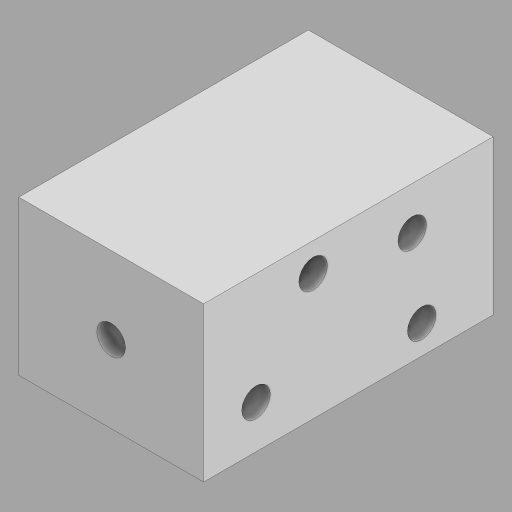
# Autodesk Inventor part: Solinoyd_telo
Saved by Autodesk Inventor 2024.2 (Build 282272000, 272)
## iProperties
Created: 2023-12-22
Part Number: Solinoyd_telo
Material: Типовые
Document SubType Name: Modeling
Designer: Fedor Orlov
Density: 1 g/cm^3
Appearance: По умолчанию
Author: Fedor Orlov
Autodesk Inventor part; units mm, degrees
ref_plane "YZ Plane" through (0, 0, 0) normal (1, 0, 0) x (0, 1, 0)
ref_plane "XZ Plane" through (0, 0, 0) normal (0, 1, 0) x (-1, 0, 0)
ref_plane "XY Plane" through (0, 0, 0) normal (0, 0, 1) x (1, 0, 0)
sketch "Эскиз1" plane through (0, 0, 0) normal (0, 1, 0) x (-1, 0, 0)
  line L0 (-9.7, -15.2) -> (9.7, -15.2)
  line L1 (9.7, -15.2) -> (9.7, 15.2)
  line L2 (9.7, 15.2) -> (-9.7, 15.2)
  line L3 (-9.7, 15.2) -> (-9.7, -15.2)
  line L4 (-9.7, -15.2) -> (9.7, 15.2) construction
  line L5 (9.7, -15.2) -> (-9.7, 15.2) construction
  point P0 (0, 0)
  dimension "d0" = 30.4
  dimension "d1" = 19.4
  constraints: 12 end point, 2 midpoint, 2 parallel, 1 horizontal, 1 perpendicular
  measures "d0" distance of L0.end L1.end
  measures "d1" distance of L1.end L2.end
extrude "Выдавливание1" add sketch "Эскиз1" along normal blind 16.2
sketch "Эскиз2" plane through (9.7, 0, -15.2) normal (0, 0, -1) x (-1, 0, 0)
  line L0 (19.4, 16.2) -> (0, 16.2) projected
  line L1 (19.4, 0) -> (19.4, 16.2) projected
  line L2 (0, 16.2) -> (19.4, 0) construction
  line L3 (19.4, 0) -> (0, 0) projected
  line L4 (19.4, 16.2) -> (0, 0) construction
  circle A0 centre (9.7, 8.1) radius 1.5
  point P0 (9.7, 0)
  dimension "d4" = 3
  constraints: 4 end point, 1 centre point, 1 midpoint
  measures "d4" diameter of A0
extrude "Выдавливание2" cut sketch "Эскиз2" against normal through all
sketch "Эскиз3" plane through (9.7, 0, 15.2) normal (1, 0, 0) x (0, 0, -1)
  circle A0 centre (21.9, 11.7) radius 1.5
  line L0 (0, 16.2) -> (30.4, 16.2) projected
  line L1 (30.4, 0) -> (30.4, 16.2) projected
  circle A1 centre (5.5, 4.5) radius 1.5
  circle A2 centre (22.9, 3) radius 1.5
  circle A3 centre (11.5, 13.2) radius 1.5
  line L2 (0, 0) -> (30.4, 0) projected
  line L3 (0, 0) -> (0, 16.2) projected
  point P0 (15.2, 0)
  dimension "d7" = 3
  dimension "d8" = 4.5
  dimension "d9" = 8.5
  dimension "d10" = 3
  dimension "d11" = 3
  dimension "d12" = 3
  dimension "d13" = 4.5
  dimension "d14" = 3
  dimension "d15" = 3
  dimension "d16" = 7.5
  dimension "d17" = 5.5
  dimension "d18" = 11.5
  constraints: 4 centre point
  measures "d7" diameter of A0
  measures "d8" distance from line of L0 A0.centre
  measures "d9" distance from line of L1 A0.centre
  measures "d10" diameter of A1
  measures "d11" diameter of A2
  measures "d12" diameter of A3
  measures "d13" distance from line of L2 A1.centre
  measures "d14" distance from line of L2 A2.centre
  measures "d15" distance from line of L0 A3.centre
  measures "d16" distance from line of L1 A2.centre
  measures "d17" distance from line of L3 A1.centre
  measures "d18" distance from line of L3 A3.centre
extrude "Выдавливание3" cut sketch "Эскиз3" against normal blind 3.5 contours A0 | A1 | A2 | A3
sketch "Эскиз4" plane through (9.7, 0, -15.2) normal (0, 0, -1) x (-1, 0, 0)
  line L0 (16.2554, 14.2612) -> (16.2554, 1.9388) construction
  line L1 (16.2554, 1.9388) -> (12.5446, 1.9388) construction
  line L2 (12.5446, 1.9388) -> (12.5446, 14.2612) construction
  line L3 (12.5446, 14.2612) -> (16.2554, 14.2612) construction
  line L4 (16.2554, 1.9388) -> (12.5446, 14.2612) construction
  line L5 (16.2554, 14.2612) -> (12.5446, 1.9388) construction
  circle A0 centre (9.7, 8.1) radius 1.5 projected
  line L6 (0, 0) -> (0, 16.2) projected
  line L7 (0, 8.1) -> (19.4, 8.1) construction
  line L8 (19.4, 0) -> (19.4, 16.2) projected
  line L9 (13.2074, 11.7393) -> (13.2074, 12.1444)
  line L10 (13.2074, 12.1444) -> (15.8947, 12.1444)
  line L11 (15.8947, 12.1444) -> (15.8947, 13.5473)
  line L12 (15.8947, 13.5473) -> (13.2074, 13.5473)
  line L13 (13.2074, 13.5473) -> (13.2074, 13.9524)
  line L14 (13.2074, 13.9524) -> (16.2554, 13.9524)
  line L15 (16.2554, 13.9524) -> (16.2554, 11.7393)
  line L16 (16.2554, 11.7393) -> (13.2074, 11.7393)
  spline S0 degree 2 poles (13.1555, 10.1585) (13.1555, 10.7068) (13.7705, 11.3095) (14.3386, 11.3095) knots 0 0 0 1 2 2 2
  spline S1 degree 2 poles (14.3386, 11.3095) (14.8969, 11.3095) (15.5588, 10.7241) (15.5588, 10.2523) knots 0 0 0 1 2 2 2
  spline S2 degree 2 poles (15.5588, 10.2523) (15.5588, 10.0399) (15.4353, 9.7114) (15.3044, 9.5904) knots 0 0 0 1 2 2 2
  spline S3 degree 2 poles (15.3044, 9.5904) (15.1735, 9.4669) (14.7956, 9.336) (14.5214, 9.336) knots 0 0 0 1 2 2 2
  line L17 (14.5214, 9.336) -> (14.3115, 9.336)
  line L18 (14.3115, 9.336) -> (14.3115, 10.9193)
  spline S4 degree 2 poles (14.3115, 10.9193) (13.9138, 10.9193) (13.4914, 10.5191) (13.4914, 10.1634) knots 0 0 0 1 2 2 2
  spline S5 degree 2 poles (13.4914, 10.1634) (13.4914, 10.0375) (13.5482, 9.7929) (13.5927, 9.6941) knots 0 0 0 1 2 2 2
  spline S6 degree 2 poles (13.5927, 9.6941) (13.6421, 9.5904) (13.7285, 9.4471) (13.7681, 9.4002) knots 0 0 0 1 2 2 2
  line L19 (13.7681, 9.4002) -> (13.7681, 9.378)
  line L20 (13.7681, 9.378) -> (13.3482, 9.378)
  spline S7 degree 2 poles (13.3482, 9.378) (13.321, 9.4447) (13.2419, 9.6472) (13.2197, 9.7262) knots 0 0 0 1 2 2 2
  spline S8 degree 2 poles (13.2197, 9.7262) (13.1876, 9.8374) (13.1555, 10.0202) (13.1555, 10.1585) knots 0 0 0 1 2 2 2
  spline S9 degree 2 poles (14.6054, 9.7114) (14.761, 9.7164) (14.9882, 9.7806) (15.0648, 9.8423) knots 0 0 0 1 2 2 2
  spline S10 degree 2 poles (15.0648, 9.8423) (15.1513, 9.909) (15.2427, 10.119) (15.2427, 10.2746) knots 0 0 0 1 2 2 2
  spline S11 degree 2 poles (15.2427, 10.2746) (15.2427, 10.4277) (15.1513, 10.6426) (15.0623, 10.7315) knots 0 0 0 1 2 2 2
  spline S12 degree 2 poles (15.0623, 10.7315) (14.971, 10.818) (14.7511, 10.9069) (14.6054, 10.9193) knots 0 0 0 1 2 2 2
  line L21 (14.6054, 10.9193) -> (14.6054, 9.7114)
  line L22 (13.2074, 7.1426) -> (13.2074, 7.5279)
  line L23 (13.2074, 7.5279) -> (15.1636, 7.5279)
  line L24 (15.1636, 7.5279) -> (15.1636, 8.5604)
  line L25 (15.1636, 8.5604) -> (13.2074, 8.5604)
  line L26 (13.2074, 8.5604) -> (13.2074, 8.9457)
  line L27 (13.2074, 8.9457) -> (15.4946, 8.9457)
  line L28 (15.4946, 8.9457) -> (15.4946, 7.1426)
  line L29 (15.4946, 7.1426) -> (13.2074, 7.1426)
  spline S13 degree 2 poles (13.1555, 5.5914) (13.1555, 6.1398) (13.7705, 6.7425) (14.3386, 6.7425) knots 0 0 0 1 2 2 2
  spline S14 degree 2 poles (14.3386, 6.7425) (14.8969, 6.7425) (15.5588, 6.1571) (15.5588, 5.6853) knots 0 0 0 1 2 2 2
  spline S15 degree 2 poles (15.5588, 5.6853) (15.5588, 5.4729) (15.4353, 5.1444) (15.3044, 5.0233) knots 0 0 0 1 2 2 2
  spline S16 degree 2 poles (15.3044, 5.0233) (15.1735, 4.8998) (14.7956, 4.7689) (14.5214, 4.7689) knots 0 0 0 1 2 2 2
  line L30 (14.5214, 4.7689) -> (14.3115, 4.7689)
  line L31 (14.3115, 4.7689) -> (14.3115, 6.3522)
  spline S17 degree 2 poles (14.3115, 6.3522) (13.9138, 6.3522) (13.4914, 5.952) (13.4914, 5.5964) knots 0 0 0 1 2 2 2
  spline S18 degree 2 poles (13.4914, 5.5964) (13.4914, 5.4704) (13.5482, 5.2259) (13.5927, 5.1271) knots 0 0 0 1 2 2 2
  spline S19 degree 2 poles (13.5927, 5.1271) (13.6421, 5.0233) (13.7285, 4.8801) (13.7681, 4.8331) knots 0 0 0 1 2 2 2
  line L32 (13.7681, 4.8331) -> (13.7681, 4.8109)
  line L33 (13.7681, 4.8109) -> (13.3482, 4.8109)
  spline S20 degree 2 poles (13.3482, 4.8109) (13.321, 4.8776) (13.2419, 5.0801) (13.2197, 5.1592) knots 0 0 0 1 2 2 2
  spline S21 degree 2 poles (13.2197, 5.1592) (13.1876, 5.2703) (13.1555, 5.4531) (13.1555, 5.5914) knots 0 0 0 1 2 2 2
  spline S22 degree 2 poles (14.6054, 5.1444) (14.761, 5.1493) (14.9882, 5.2135) (15.0648, 5.2753) knots 0 0 0 1 2 2 2
  spline S23 degree 2 poles (15.0648, 5.2753) (15.1513, 5.342) (15.2427, 5.5519) (15.2427, 5.7075) knots 0 0 0 1 2 2 2
  spline S24 degree 2 poles (15.2427, 5.7075) (15.2427, 5.8607) (15.1513, 6.0755) (15.0623, 6.1645) knots 0 0 0 1 2 2 2
  spline S25 degree 2 poles (15.0623, 6.1645) (14.971, 6.2509) (14.7511, 6.3398) (14.6054, 6.3522) knots 0 0 0 1 2 2 2
  line L34 (14.6054, 6.3522) -> (14.6054, 5.1444)
  line L35 (12.659, 2.4199) -> (12.659, 2.7781)
  line L36 (12.659, 2.7781) -> (13.2123, 2.7781)
  line L37 (13.2123, 2.7781) -> (13.2123, 4.2823)
  line L38 (13.2123, 4.2823) -> (12.659, 4.2823)
  line L39 (12.659, 4.2823) -> (12.659, 4.6405)
  line L40 (12.659, 4.6405) -> (13.5359, 4.6405)
  line L41 (13.5359, 4.6405) -> (13.5359, 4.4898)
  spline S26 degree 2 poles (13.5359, 4.4898) (13.8545, 4.2947) (14.8845, 4.0477) (15.4946, 4.0477) knots 0 0 0 1 2 2 2
  line L42 (15.4946, 4.0477) -> (15.4946, 2.6472)
  line L43 (15.4946, 2.6472) -> (13.5359, 2.6472)
  line L44 (13.5359, 2.6472) -> (13.5359, 2.4199)
  line L45 (13.5359, 2.4199) -> (12.659, 2.4199)
  line L46 (13.5359, 3.0325) -> (15.171, 3.0325)
  line L47 (15.171, 3.0325) -> (15.171, 3.6846)
  spline S27 degree 2 poles (15.171, 3.6846) (14.6597, 3.7117) (13.815, 3.939) (13.5359, 4.1119) knots 0 0 0 1 2 2 2
  line L48 (13.5359, 4.1119) -> (13.5359, 3.0325)
  point P0 (9.7, 0)
  point P1 (14.4, 8.1)
  point P2 (14.4, 8.1)
  dimension "d21" = 5
  constraints: 6 end point, 4 midpoint, 1 point on line, 2 other
  measures "d21" distance from line of L8 point (14.4, 8.1)
extrude "Выдавливание4" cut sketch "Эскиз4" against normal blind 0.2 contours L9 L10 L11 L12 L13 L14 L15 L16 | S0 S1 S2 S3 L17 L18 S4 S5 S6 L19 L20 S7 S8 | L22 L23 L24 L25 L26 L27 L28 L29 | S13 S14 S15 S16 L30 L31 S17 S18 S19 L32 L33 S20 S21 | L35 L36 L37 L38 L39 L40 L41 S26 L42 L43 L44 L45
sketch "Эскиз5" plane through (-9.7, 0, -15.2) normal (-1, 0, 0) x (0, 0, 1)
  line L0 (9.6722, 9.7186) -> (20.6663, 9.7186) construction
  line L1 (20.6663, 9.7186) -> (20.6663, 6.5249) construction
  line L2 (20.6663, 6.5249) -> (9.6722, 6.5249) construction
  line L3 (9.6722, 6.5249) -> (9.6722, 9.7186) construction
  line L4 (20.6663, 9.7186) -> (9.6722, 6.5249) construction
  line L5 (20.6663, 6.5249) -> (9.6722, 9.7186) construction
  line L6 (30.4, 0) -> (30.4, 16.2) projected
  line L7 (0, 0) -> (0, 16.2) projected
  line L8 (30.4, 16.2) -> (0, 0) construction
  line L9 (0, 16.2) -> (30.4, 16.2) projected
  line L10 (0, 0) -> (30.4, 0) projected
  line L11 (0, 16.2) -> (30.4, 0) construction
  spline S0 degree 2 poles (11.7446, 8.0587) (11.7446, 7.8933) (11.6186, 7.6364) (11.5075, 7.5524) knots 0 0 0 1 2 2 2
  spline S1 degree 2 poles (11.5075, 7.5524) (11.3691, 7.4437) (11.0629, 7.3671) (10.8504, 7.3671) knots 0 0 0 1 2 2 2
  line L12 (10.8504, 7.3671) -> (9.9513, 7.3671)
  line L13 (9.9513, 7.3671) -> (9.9513, 9.6544)
  line L14 (9.9513, 9.6544) -> (10.7912, 9.6544)
  spline S2 degree 2 poles (10.7912, 9.6544) (11.0431, 9.6544) (11.2753, 9.6247) (11.3914, 9.5605) knots 0 0 0 1 2 2 2
  spline S3 degree 2 poles (11.3914, 9.5605) (11.5124, 9.4938) (11.626, 9.2765) (11.626, 9.1283) knots 0 0 0 1 2 2 2
  spline S4 degree 2 poles (11.626, 9.1283) (11.626, 8.9652) (11.4457, 8.7034) (11.2975, 8.6318) knots 0 0 0 1 2 2 2
  line L15 (11.2975, 8.6318) -> (11.3074, 8.6194)
  spline S5 degree 2 poles (11.3074, 8.6194) (11.4926, 8.57) (11.7446, 8.2835) (11.7446, 8.0587) knots 0 0 0 1 2 2 2
  spline S6 degree 2 poles (11.3469, 8.0563) (11.3469, 8.1748) (11.2802, 8.3156) (11.1641, 8.37) knots 0 0 0 1 2 2 2
  spline S7 degree 2 poles (11.1641, 8.37) (11.0925, 8.4045) (10.9295, 8.4218) (10.7837, 8.4218) knots 0 0 0 1 2 2 2
  line L16 (10.7837, 8.4218) -> (10.3317, 8.4218)
  line L17 (10.3317, 8.4218) -> (10.3317, 7.6734)
  line L18 (10.3317, 7.6734) -> (10.6652, 7.6734)
  spline S8 degree 2 poles (10.6652, 7.6734) (10.8727, 7.6734) (11.1024, 7.7055) (11.1839, 7.7549) knots 0 0 0 1 2 2 2
  spline S9 degree 2 poles (11.1839, 7.7549) (11.2703, 7.8093) (11.3469, 7.9476) (11.3469, 8.0563) knots 0 0 0 1 2 2 2
  spline S10 degree 2 poles (11.2283, 9.069) (11.2283, 9.148) (11.1765, 9.2616) (11.1147, 9.2938) knots 0 0 0 1 2 2 2
  spline S11 degree 2 poles (11.1147, 9.2938) (11.0406, 9.3333) (10.8578, 9.3481) (10.6973, 9.3481) knots 0 0 0 1 2 2 2
  line L19 (10.6973, 9.3481) -> (10.3317, 9.3481)
  line L20 (10.3317, 9.3481) -> (10.3317, 8.7207)
  line L21 (10.3317, 8.7207) -> (10.7739, 8.7207)
  spline S12 degree 2 poles (10.7739, 8.7207) (10.9147, 8.7207) (11.0332, 8.7479) (11.1048, 8.7899) knots 0 0 0 1 2 2 2
  spline S13 degree 2 poles (11.1048, 8.7899) (11.1715, 8.8319) (11.2283, 8.9702) (11.2283, 9.069) knots 0 0 0 1 2 2 2
  spline S14 degree 2 poles (13.9429, 8.0587) (13.9429, 7.8933) (13.8169, 7.6364) (13.7058, 7.5524) knots 0 0 0 1 2 2 2
  spline S15 degree 2 poles (13.7058, 7.5524) (13.5675, 7.4437) (13.2612, 7.3671) (13.0488, 7.3671) knots 0 0 0 1 2 2 2
  line L22 (13.0488, 7.3671) -> (12.1497, 7.3671)
  line L23 (12.1497, 7.3671) -> (12.1497, 9.6544)
  line L24 (12.1497, 9.6544) -> (12.9895, 9.6544)
  spline S16 degree 2 poles (12.9895, 9.6544) (13.2414, 9.6544) (13.4736, 9.6247) (13.5897, 9.5605) knots 0 0 0 1 2 2 2
  spline S17 degree 2 poles (13.5897, 9.5605) (13.7107, 9.4938) (13.8243, 9.2765) (13.8243, 9.1283) knots 0 0 0 1 2 2 2
  spline S18 degree 2 poles (13.8243, 9.1283) (13.8243, 8.9652) (13.644, 8.7034) (13.4958, 8.6318) knots 0 0 0 1 2 2 2
  line L25 (13.4958, 8.6318) -> (13.5057, 8.6194)
  spline S19 degree 2 poles (13.5057, 8.6194) (13.691, 8.57) (13.9429, 8.2835) (13.9429, 8.0587) knots 0 0 0 1 2 2 2
  spline S20 degree 2 poles (13.5452, 8.0563) (13.5452, 8.1748) (13.4785, 8.3156) (13.3624, 8.37) knots 0 0 0 1 2 2 2
  spline S21 degree 2 poles (13.3624, 8.37) (13.2908, 8.4045) (13.1278, 8.4218) (12.9821, 8.4218) knots 0 0 0 1 2 2 2
  line L26 (12.9821, 8.4218) -> (12.53, 8.4218)
  line L27 (12.53, 8.4218) -> (12.53, 7.6734)
  line L28 (12.53, 7.6734) -> (12.8635, 7.6734)
  spline S22 degree 2 poles (12.8635, 7.6734) (13.071, 7.6734) (13.3007, 7.7055) (13.3822, 7.7549) knots 0 0 0 1 2 2 2
  spline S23 degree 2 poles (13.3822, 7.7549) (13.4687, 7.8093) (13.5452, 7.9476) (13.5452, 8.0563) knots 0 0 0 1 2 2 2
  spline S24 degree 2 poles (13.4267, 9.069) (13.4267, 9.148) (13.3748, 9.2616) (13.313, 9.2938) knots 0 0 0 1 2 2 2
  spline S25 degree 2 poles (13.313, 9.2938) (13.2389, 9.3333) (13.0562, 9.3481) (12.8956, 9.3481) knots 0 0 0 1 2 2 2
  line L29 (12.8956, 9.3481) -> (12.53, 9.3481)
  line L30 (12.53, 9.3481) -> (12.53, 8.7207)
  line L31 (12.53, 8.7207) -> (12.9722, 8.7207)
  spline S26 degree 2 poles (12.9722, 8.7207) (13.113, 8.7207) (13.2315, 8.7479) (13.3032, 8.7899) knots 0 0 0 1 2 2 2
  spline S27 degree 2 poles (13.3032, 8.7899) (13.3699, 8.8319) (13.4267, 8.9702) (13.4267, 9.069) knots 0 0 0 1 2 2 2
  spline S28 degree 2 poles (15.3409, 7.3153) (14.7926, 7.3153) (14.1899, 7.9303) (14.1899, 8.4984) knots 0 0 0 1 2 2 2
  spline S29 degree 2 poles (14.1899, 8.4984) (14.1899, 9.0566) (14.7753, 9.7186) (15.2471, 9.7186) knots 0 0 0 1 2 2 2
  spline S30 degree 2 poles (15.2471, 9.7186) (15.4595, 9.7186) (15.788, 9.5951) (15.909, 9.4642) knots 0 0 0 1 2 2 2
  spline S31 degree 2 poles (15.909, 9.4642) (16.0325, 9.3333) (16.1634, 8.9554) (16.1634, 8.6812) knots 0 0 0 1 2 2 2
  line L32 (16.1634, 8.6812) -> (16.1634, 8.4712)
  line L33 (16.1634, 8.4712) -> (14.5802, 8.4712)
  spline S32 degree 2 poles (14.5802, 8.4712) (14.5802, 8.0736) (14.9803, 7.6512) (15.336, 7.6512) knots 0 0 0 1 2 2 2
  spline S33 degree 2 poles (15.336, 7.6512) (15.462, 7.6512) (15.7065, 7.708) (15.8053, 7.7525) knots 0 0 0 1 2 2 2
  spline S34 degree 2 poles (15.8053, 7.7525) (15.909, 7.8019) (16.0523, 7.8883) (16.0992, 7.9278) knots 0 0 0 1 2 2 2
  line L34 (16.0992, 7.9278) -> (16.1215, 7.9278)
  line L35 (16.1215, 7.9278) -> (16.1215, 7.5079)
  spline S35 degree 2 poles (16.1215, 7.5079) (16.0548, 7.4808) (15.8522, 7.4017) (15.7732, 7.3795) knots 0 0 0 1 2 2 2
  spline S36 degree 2 poles (15.7732, 7.3795) (15.662, 7.3474) (15.4792, 7.3153) (15.3409, 7.3153) knots 0 0 0 1 2 2 2
  spline S37 degree 2 poles (15.788, 8.7652) (15.7831, 8.9208) (15.7188, 9.148) (15.6571, 9.2246) knots 0 0 0 1 2 2 2
  spline S38 degree 2 poles (15.6571, 9.2246) (15.5904, 9.311) (15.3804, 9.4024) (15.2248, 9.4024) knots 0 0 0 1 2 2 2
  spline S39 degree 2 poles (15.2248, 9.4024) (15.0717, 9.4024) (14.8568, 9.311) (14.7679, 9.2221) knots 0 0 0 1 2 2 2
  spline S40 degree 2 poles (14.7679, 9.2221) (14.6814, 9.1307) (14.5925, 8.9109) (14.5802, 8.7652) knots 0 0 0 1 2 2 2
  line L36 (14.5802, 8.7652) -> (15.788, 8.7652)
  spline S41 degree 2 poles (18.4704, 8.5725) (18.4704, 7.9995) (17.9246, 7.3227) (17.5071, 7.3227) knots 0 0 0 1 2 2 2
  spline S42 degree 2 poles (17.5071, 7.3227) (17.3367, 7.3227) (17.0749, 7.4017) (16.939, 7.4832) knots 0 0 0 1 2 2 2
  line L37 (16.939, 7.4832) -> (16.939, 6.5249)
  line L38 (16.939, 6.5249) -> (16.5537, 6.5249)
  line L39 (16.5537, 6.5249) -> (16.5537, 9.6544)
  line L40 (16.5537, 9.6544) -> (16.939, 9.6544)
  line L41 (16.939, 9.6544) -> (16.939, 9.4148)
  spline S43 degree 2 poles (16.939, 9.4148) (17.0823, 9.5457) (17.433, 9.7186) (17.638, 9.7186) knots 0 0 0 1 2 2 2
  spline S44 degree 2 poles (17.638, 9.7186) (18.0308, 9.7186) (18.4704, 9.0962) (18.4704, 8.5725) knots 0 0 0 1 2 2 2
  spline S45 degree 2 poles (18.0728, 8.528) (18.0728, 8.9208) (17.8233, 9.353) (17.5442, 9.353) knots 0 0 0 1 2 2 2
  spline S46 degree 2 poles (17.5442, 9.353) (17.3812, 9.353) (17.0749, 9.2073) (16.939, 9.0937) knots 0 0 0 1 2 2 2
  line L42 (16.939, 9.0937) -> (16.939, 7.7945)
  spline S47 degree 2 poles (16.939, 7.7945) (17.0897, 7.7228) (17.3046, 7.6685) (17.4429, 7.6685) knots 0 0 0 1 2 2 2
  spline S48 degree 2 poles (17.4429, 7.6685) (17.7418, 7.6685) (18.0728, 8.1081) (18.0728, 8.528) knots 0 0 0 1 2 2 2
  line L43 (20.6465, 7.3671) -> (20.1747, 7.3671)
  line L44 (20.1747, 7.3671) -> (19.619, 8.2267)
  line L45 (19.619, 8.2267) -> (19.0484, 7.3671)
  line L46 (19.0484, 7.3671) -> (18.6112, 7.3671)
  line L47 (18.6112, 7.3671) -> (19.4041, 8.5009)
  line L48 (19.4041, 8.5009) -> (18.6186, 9.6544)
  line L49 (18.6186, 9.6544) -> (19.0904, 9.6544)
  line L50 (19.0904, 9.6544) -> (19.6437, 8.8022)
  line L51 (19.6437, 8.8022) -> (20.2093, 9.6544)
  line L52 (20.2093, 9.6544) -> (20.6465, 9.6544)
  line L53 (20.6465, 9.6544) -> (19.8586, 8.5256)
  line L54 (19.8586, 8.5256) -> (20.6465, 7.3671)
  point P0 (15.2, 0)
  constraints: 8 end point, 2 other
extrude "Выдавливание5" cut sketch "Эскиз5" against normal blind 0.2 contours S0 S1 L12 L13 L14 S2 S3 S4 L15 S5 | S14 S15 L22 L23 L24 S16 S17 S18 L25 S19 | S28 S29 S30 S31 L32 L33 S32 S33 S34 L34 L35 S35 S36 | S41 S42 L37 L38 L39 L40 L41 S43 S44 | L43 L44 L45 L46 L47 L48 L49 L50 L51 L52 L53 L54
equation "\"d14\" = d15"
